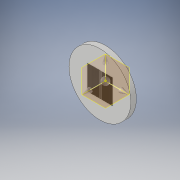
# Autodesk Inventor part: mask
Saved by Autodesk Inventor 2018 (Build 220112000, 112)
## iProperties
Created: 2019-06-01
Part Number: mask
Material: Generic
Document SubType Name: Modeling
Designer: 3esha
Density: 1 g/cm^3
Appearance: Default
Author: 3esha
Autodesk Inventor part; units mm, degrees
ref_plane "YZ Plane" through (0, 0, 0) normal (1, 0, 0) x (0, 1, 0)
ref_plane "XZ Plane" through (0, 0, 0) normal (0, 1, 0) x (-1, 0, 0)
ref_plane "XY Plane" through (0, 0, 0) normal (0, 0, 1) x (1, 0, 0)
sketch "Sketch9" plane through (0, 0, 0) normal (0, 0, 1) x (1, 0, 0)
  circle A0 centre (0, 0) radius 12.7
  line L0 (-0.3556, 4.953) -> (-0.4826, 4.953)
  line L1 (-0.4826, 4.953) -> (-0.4826, -5.0546)
  line L2 (-0.4826, -5.0546) -> (-0.3556, -5.0546)
  line L3 (-0.3556, -5.0546) -> (-0.3556, 4.953)
  line L4 (-0.635, 4.953) -> (-0.762, 4.953)
  line L5 (-0.762, 4.953) -> (-0.762, -5.0546)
  line L6 (-0.762, -5.0546) -> (-0.635, -5.0546)
  line L7 (-0.635, -5.0546) -> (-0.635, 4.953)
  line L8 (-0.889, 4.953) -> (-1.0414, 4.953)
  line L9 (-1.0414, 4.953) -> (-1.0414, -5.0546)
  line L10 (-1.0414, -5.0546) -> (-0.889, -5.0546)
  line L11 (-0.889, -5.0546) -> (-0.889, 4.953)
  line L12 (-1.1684, 4.953) -> (-1.2954, 4.953)
  line L13 (-1.2954, 4.953) -> (-1.2954, -5.0546)
  line L14 (-1.2954, -5.0546) -> (-1.1684, -5.0546)
  line L15 (-1.1684, -5.0546) -> (-1.1684, 4.953)
  line L16 (-1.4224, 4.953) -> (-1.5748, 4.953)
  line L17 (-1.5748, 4.953) -> (-1.5748, -5.0546)
  line L18 (-1.5748, -5.0546) -> (-1.4224, -5.0546)
  line L19 (-1.4224, -5.0546) -> (-1.4224, 4.953)
  line L20 (-1.7018, 4.953) -> (-1.8288, 4.953)
  line L21 (-1.8288, 4.953) -> (-1.8288, -5.0546)
  line L22 (-1.8288, -5.0546) -> (-1.7018, -5.0546)
  line L23 (-1.7018, -5.0546) -> (-1.7018, 4.953)
  line L24 (-1.9812, 4.953) -> (-2.1082, 4.953)
  line L25 (-2.1082, 4.953) -> (-2.1082, -5.0546)
  line L26 (-2.1082, -5.0546) -> (-1.9812, -5.0546)
  line L27 (-1.9812, -5.0546) -> (-1.9812, 4.953)
  line L28 (-2.2352, 4.953) -> (-2.3876, 4.953)
  line L29 (-2.3876, 4.953) -> (-2.3876, -5.0546)
  line L30 (-2.3876, -5.0546) -> (-2.2352, -5.0546)
  line L31 (-2.2352, -5.0546) -> (-2.2352, 4.953)
  line L32 (-2.5146, 4.953) -> (-2.6416, 4.953)
  line L33 (-2.6416, 4.953) -> (-2.6416, -5.0546)
  line L34 (-2.6416, -5.0546) -> (-2.5146, -5.0546)
  line L35 (-2.5146, -5.0546) -> (-2.5146, 4.953)
  line L36 (-2.794, 4.953) -> (-2.921, 4.953)
  line L37 (-2.921, 4.953) -> (-2.921, -5.0546)
  line L38 (-2.921, -5.0546) -> (-2.794, -5.0546)
  line L39 (-2.794, -5.0546) -> (-2.794, 4.953)
  line L40 (-3.048, 4.953) -> (-3.2004, 4.953)
  line L41 (-3.2004, 4.953) -> (-3.2004, -5.0546)
  line L42 (-3.2004, -5.0546) -> (-3.048, -5.0546)
  line L43 (-3.048, -5.0546) -> (-3.048, 4.953)
  line L44 (-3.3274, 4.953) -> (-3.4544, 4.953)
  line L45 (-3.4544, 4.953) -> (-3.4544, -5.0546)
  line L46 (-3.4544, -5.0546) -> (-3.3274, -5.0546)
  line L47 (-3.3274, -5.0546) -> (-3.3274, 4.953)
  line L48 (-3.6068, 4.953) -> (-3.7338, 4.953)
  line L49 (-3.7338, 4.953) -> (-3.7338, -5.0546)
  line L50 (-3.7338, -5.0546) -> (-3.6068, -5.0546)
  line L51 (-3.6068, -5.0546) -> (-3.6068, 4.953)
  line L52 (-3.8608, 4.953) -> (-3.9878, 4.953)
  line L53 (-3.9878, 4.953) -> (-3.9878, -5.0546)
  line L54 (-3.9878, -5.0546) -> (-3.8608, -5.0546)
  line L55 (-3.8608, -5.0546) -> (-3.8608, 4.953)
  line L56 (-4.1402, 4.953) -> (-4.2672, 4.953)
  line L57 (-4.2672, 4.953) -> (-4.2672, -5.0546)
  line L58 (-4.2672, -5.0546) -> (-4.1402, -5.0546)
  line L59 (-4.1402, -5.0546) -> (-4.1402, 4.953)
  line L60 (-4.3942, 4.953) -> (-4.5466, 4.953)
  line L61 (-4.5466, 4.953) -> (-4.5466, -5.0546)
  line L62 (-4.5466, -5.0546) -> (-4.3942, -5.0546)
  line L63 (-4.3942, -5.0546) -> (-4.3942, 4.953)
  line L64 (-4.6736, 4.953) -> (-4.8006, 4.953)
  line L65 (-4.8006, 4.953) -> (-4.8006, -5.0546)
  line L66 (-4.8006, -5.0546) -> (-4.6736, -5.0546)
  line L67 (-4.6736, -5.0546) -> (-4.6736, 4.953)
  line L68 (-4.953, 4.953) -> (-5.08, 4.953)
  line L69 (-5.08, 4.953) -> (-5.08, -5.0546)
  line L70 (-5.08, -5.0546) -> (-4.953, -5.0546)
  line L71 (-4.953, -5.0546) -> (-4.953, 4.953)
  line L72 (-0.0762, 4.953) -> (-0.2286, 4.953)
  line L73 (-0.2286, 4.953) -> (-0.2286, -5.0546)
  line L74 (-0.2286, -5.0546) -> (-0.0762, -5.0546)
  line L75 (-0.0762, -5.0546) -> (-0.0762, 4.953)
  line L76 (0.1778, 4.953) -> (0.3302, 4.953)
  line L77 (0.3302, 4.953) -> (0.3302, -5.0546)
  line L78 (0.3302, -5.0546) -> (0.1778, -5.0546)
  line L79 (0.1778, -5.0546) -> (0.1778, 4.953)
  line L80 (5.0546, 4.953) -> (5.1816, 4.953)
  line L81 (5.1816, 4.953) -> (5.1816, -5.0546)
  line L82 (5.1816, -5.0546) -> (5.0546, -5.0546)
  line L83 (5.0546, -5.0546) -> (5.0546, 4.953)
  line L84 (4.7752, 4.953) -> (4.9022, 4.953)
  line L85 (4.9022, 4.953) -> (4.9022, -5.0546)
  line L86 (4.9022, -5.0546) -> (4.7752, -5.0546)
  line L87 (4.7752, -5.0546) -> (4.7752, 4.953)
  line L88 (4.4958, 4.953) -> (4.6482, 4.953)
  line L89 (4.6482, 4.953) -> (4.6482, -5.0546)
  line L90 (4.6482, -5.0546) -> (4.4958, -5.0546)
  line L91 (4.4958, -5.0546) -> (4.4958, 4.953)
  line L92 (4.2418, 4.953) -> (4.3688, 4.953)
  line L93 (4.3688, 4.953) -> (4.3688, -5.0546)
  line L94 (4.3688, -5.0546) -> (4.2418, -5.0546)
  line L95 (4.2418, -5.0546) -> (4.2418, 4.953)
  line L96 (3.9624, 4.953) -> (4.0894, 4.953)
  line L97 (4.0894, 4.953) -> (4.0894, -5.0546)
  line L98 (4.0894, -5.0546) -> (3.9624, -5.0546)
  line L99 (3.9624, -5.0546) -> (3.9624, 4.953)
  line L100 (3.7084, 4.953) -> (3.8354, 4.953)
  line L101 (3.8354, 4.953) -> (3.8354, -5.0546)
  line L102 (3.8354, -5.0546) -> (3.7084, -5.0546)
  line L103 (3.7084, -5.0546) -> (3.7084, 4.953)
  line L104 (3.429, 4.953) -> (3.556, 4.953)
  line L105 (3.556, 4.953) -> (3.556, -5.0546)
  line L106 (3.556, -5.0546) -> (3.429, -5.0546)
  line L107 (3.429, -5.0546) -> (3.429, 4.953)
  line L108 (3.1496, 4.953) -> (3.302, 4.953)
  line L109 (3.302, 4.953) -> (3.302, -5.0546)
  line L110 (3.302, -5.0546) -> (3.1496, -5.0546)
  line L111 (3.1496, -5.0546) -> (3.1496, 4.953)
  line L112 (2.8956, 4.953) -> (3.0226, 4.953)
  line L113 (3.0226, 4.953) -> (3.0226, -5.0546)
  line L114 (3.0226, -5.0546) -> (2.8956, -5.0546)
  line L115 (2.8956, -5.0546) -> (2.8956, 4.953)
  line L116 (2.6162, 4.953) -> (2.7432, 4.953)
  line L117 (2.7432, 4.953) -> (2.7432, -5.0546)
  line L118 (2.7432, -5.0546) -> (2.6162, -5.0546)
  line L119 (2.6162, -5.0546) -> (2.6162, 4.953)
  line L120 (2.3368, 4.953) -> (2.4892, 4.953)
  line L121 (2.4892, 4.953) -> (2.4892, -5.0546)
  line L122 (2.4892, -5.0546) -> (2.3368, -5.0546)
  line L123 (2.3368, -5.0546) -> (2.3368, 4.953)
  line L124 (2.0828, 4.953) -> (2.2098, 4.953)
  line L125 (2.2098, 4.953) -> (2.2098, -5.0546)
  line L126 (2.2098, -5.0546) -> (2.0828, -5.0546)
  line L127 (2.0828, -5.0546) -> (2.0828, 4.953)
  line L128 (1.8034, 4.953) -> (1.9304, 4.953)
  line L129 (1.9304, 4.953) -> (1.9304, -5.0546)
  line L130 (1.9304, -5.0546) -> (1.8034, -5.0546)
  line L131 (1.8034, -5.0546) -> (1.8034, 4.953)
  line L132 (1.524, 4.953) -> (1.6764, 4.953)
  line L133 (1.6764, 4.953) -> (1.6764, -5.0546)
  line L134 (1.6764, -5.0546) -> (1.524, -5.0546)
  line L135 (1.524, -5.0546) -> (1.524, 4.953)
  line L136 (1.27, 4.953) -> (1.397, 4.953)
  line L137 (1.397, 4.953) -> (1.397, -5.0546)
  line L138 (1.397, -5.0546) -> (1.27, -5.0546)
  line L139 (1.27, -5.0546) -> (1.27, 4.953)
  line L140 (0.9906, 4.953) -> (1.143, 4.953)
  line L141 (1.143, 4.953) -> (1.143, -5.0546)
  line L142 (1.143, -5.0546) -> (0.9906, -5.0546)
  line L143 (0.9906, -5.0546) -> (0.9906, 4.953)
  line L144 (0.7366, 4.953) -> (0.8636, 4.953)
  line L145 (0.8636, 4.953) -> (0.8636, -5.0546)
  line L146 (0.8636, -5.0546) -> (0.7366, -5.0546)
  line L147 (0.7366, -5.0546) -> (0.7366, 4.953)
  line L148 (0.4572, 4.953) -> (0.5842, 4.953)
  line L149 (0.5842, 4.953) -> (0.5842, -5.0546)
  line L150 (0.5842, -5.0546) -> (0.4572, -5.0546)
  line L151 (0.4572, -5.0546) -> (0.4572, 4.953)
  line L152 (-5.08, 4.953) -> (-4.953, 4.953)
  line L153 (-4.953, 4.953) -> (-4.953, -5.0546)
  line L154 (-4.953, -5.0546) -> (-5.08, -5.0546)
  line L155 (-5.08, -5.0546) -> (-5.08, 4.953)
  line L156 (-4.8006, 4.953) -> (-4.6736, 4.953)
  line L157 (-4.6736, 4.953) -> (-4.6736, -5.0546)
  line L158 (-4.6736, -5.0546) -> (-4.8006, -5.0546)
  line L159 (-4.8006, -5.0546) -> (-4.8006, 4.953)
  line L160 (-4.2672, 4.953) -> (-4.1402, 4.953)
  line L161 (-4.1402, 4.953) -> (-4.1402, -5.0546)
  line L162 (-4.1402, -5.0546) -> (-4.2672, -5.0546)
  line L163 (-4.2672, -5.0546) -> (-4.2672, 4.953)
  line L164 (-3.9878, 4.953) -> (-3.8608, 4.953)
  line L165 (-3.8608, 4.953) -> (-3.8608, -5.0546)
  line L166 (-3.8608, -5.0546) -> (-3.9878, -5.0546)
  line L167 (-3.9878, -5.0546) -> (-3.9878, 4.953)
  line L168 (-3.7338, 4.953) -> (-3.6068, 4.953)
  line L169 (-3.6068, 4.953) -> (-3.6068, -5.0546)
  line L170 (-3.6068, -5.0546) -> (-3.7338, -5.0546)
  line L171 (-3.7338, -5.0546) -> (-3.7338, 4.953)
  line L172 (-3.4544, 4.953) -> (-3.3274, 4.953)
  line L173 (-3.3274, 4.953) -> (-3.3274, -5.0546)
  line L174 (-3.3274, -5.0546) -> (-3.4544, -5.0546)
  line L175 (-3.4544, -5.0546) -> (-3.4544, 4.953)
  line L176 (-3.2004, 4.953) -> (-3.048, 4.953)
  line L177 (-3.048, 4.953) -> (-3.048, -5.0546)
  line L178 (-3.048, -5.0546) -> (-3.2004, -5.0546)
  line L179 (-3.2004, -5.0546) -> (-3.2004, 4.953)
  line L180 (-2.921, 4.953) -> (-2.794, 4.953)
  line L181 (-2.794, 4.953) -> (-2.794, -5.0546)
  line L182 (-2.794, -5.0546) -> (-2.921, -5.0546)
  line L183 (-2.921, -5.0546) -> (-2.921, 4.953)
  line L184 (-2.6416, 4.953) -> (-2.5146, 4.953)
  line L185 (-2.5146, 4.953) -> (-2.5146, -5.0546)
  line L186 (-2.5146, -5.0546) -> (-2.6416, -5.0546)
  line L187 (-2.6416, -5.0546) -> (-2.6416, 4.953)
  line L188 (-2.3876, 4.953) -> (-2.2352, 4.953)
  line L189 (-2.2352, 4.953) -> (-2.2352, -5.0546)
  line L190 (-2.2352, -5.0546) -> (-2.3876, -5.0546)
  line L191 (-2.3876, -5.0546) -> (-2.3876, 4.953)
  line L192 (-2.1082, 4.953) -> (-1.9812, 4.953)
  line L193 (-1.9812, 4.953) -> (-1.9812, -5.0546)
  line L194 (-1.9812, -5.0546) -> (-2.1082, -5.0546)
  line L195 (-2.1082, -5.0546) -> (-2.1082, 4.953)
  line L196 (-1.8288, 4.953) -> (-1.7018, 4.953)
  line L197 (-1.7018, 4.953) -> (-1.7018, -5.0546)
  line L198 (-1.7018, -5.0546) -> (-1.8288, -5.0546)
  line L199 (-1.8288, -5.0546) -> (-1.8288, 4.953)
  line L200 (-1.5748, 4.953) -> (-1.4224, 4.953)
  line L201 (-1.4224, 4.953) -> (-1.4224, -5.0546)
  line L202 (-1.4224, -5.0546) -> (-1.5748, -5.0546)
  line L203 (-1.5748, -5.0546) -> (-1.5748, 4.953)
  line L204 (-1.2954, 4.953) -> (-1.1684, 4.953)
  line L205 (-1.1684, 4.953) -> (-1.1684, -5.0546)
  line L206 (-1.1684, -5.0546) -> (-1.2954, -5.0546)
  line L207 (-1.2954, -5.0546) -> (-1.2954, 4.953)
  line L208 (-1.0414, 4.953) -> (-0.889, 4.953)
  line L209 (-0.889, 4.953) -> (-0.889, -5.0546)
  line L210 (-0.889, -5.0546) -> (-1.0414, -5.0546)
  line L211 (-1.0414, -5.0546) -> (-1.0414, 4.953)
  line L212 (-0.762, 4.953) -> (-0.635, 4.953)
  line L213 (-0.635, 4.953) -> (-0.635, -5.0546)
  line L214 (-0.635, -5.0546) -> (-0.762, -5.0546)
  line L215 (-0.762, -5.0546) -> (-0.762, 4.953)
  line L216 (-0.4826, 4.953) -> (-0.3556, 4.953)
  line L217 (-0.3556, 4.953) -> (-0.3556, -5.0546)
  line L218 (-0.3556, -5.0546) -> (-0.4826, -5.0546)
  line L219 (-0.4826, -5.0546) -> (-0.4826, 4.953)
  line L220 (-0.2286, 4.953) -> (-0.0762, 4.953)
  line L221 (-0.0762, 4.953) -> (-0.0762, -5.0546)
  line L222 (-0.0762, -5.0546) -> (-0.2286, -5.0546)
  line L223 (-0.2286, -5.0546) -> (-0.2286, 4.953)
  line L224 (0.1778, 4.953) -> (0.3302, 4.953)
  line L225 (0.3302, 4.953) -> (0.3302, -5.0546)
  line L226 (0.3302, -5.0546) -> (0.1778, -5.0546)
  line L227 (0.1778, -5.0546) -> (0.1778, 4.953)
  line L228 (0.4572, 4.953) -> (0.5842, 4.953)
  line L229 (0.5842, 4.953) -> (0.5842, -5.0546)
  line L230 (0.5842, -5.0546) -> (0.4572, -5.0546)
  line L231 (0.4572, -5.0546) -> (0.4572, 4.953)
  line L232 (0.7366, 4.953) -> (0.8636, 4.953)
  line L233 (0.8636, 4.953) -> (0.8636, -5.0546)
  line L234 (0.8636, -5.0546) -> (0.7366, -5.0546)
  line L235 (0.7366, -5.0546) -> (0.7366, 4.953)
  line L236 (0.9906, 4.953) -> (1.143, 4.953)
  line L237 (1.143, 4.953) -> (1.143, -5.0546)
  line L238 (1.143, -5.0546) -> (0.9906, -5.0546)
  line L239 (0.9906, -5.0546) -> (0.9906, 4.953)
  line L240 (1.27, 4.953) -> (1.397, 4.953)
  line L241 (1.397, 4.953) -> (1.397, -5.0546)
  line L242 (1.397, -5.0546) -> (1.27, -5.0546)
  line L243 (1.27, -5.0546) -> (1.27, 4.953)
  line L244 (1.524, 4.953) -> (1.6764, 4.953)
  line L245 (1.6764, 4.953) -> (1.6764, -5.0546)
  line L246 (1.6764, -5.0546) -> (1.524, -5.0546)
  line L247 (1.524, -5.0546) -> (1.524, 4.953)
  line L248 (1.8034, 4.953) -> (1.9304, 4.953)
  line L249 (1.9304, 4.953) -> (1.9304, -5.0546)
  line L250 (1.9304, -5.0546) -> (1.8034, -5.0546)
  line L251 (1.8034, -5.0546) -> (1.8034, 4.953)
  line L252 (2.0828, 4.953) -> (2.2098, 4.953)
  line L253 (2.2098, 4.953) -> (2.2098, -5.0546)
  line L254 (2.2098, -5.0546) -> (2.0828, -5.0546)
  line L255 (2.0828, -5.0546) -> (2.0828, 4.953)
  line L256 (2.3368, 4.953) -> (2.4892, 4.953)
  line L257 (2.4892, 4.953) -> (2.4892, -5.0546)
  line L258 (2.4892, -5.0546) -> (2.3368, -5.0546)
  line L259 (2.3368, -5.0546) -> (2.3368, 4.953)
  line L260 (2.6162, 4.953) -> (2.7432, 4.953)
  line L261 (2.7432, 4.953) -> (2.7432, -5.0546)
  line L262 (2.7432, -5.0546) -> (2.6162, -5.0546)
  line L263 (2.6162, -5.0546) -> (2.6162, 4.953)
  line L264 (2.8956, 4.953) -> (3.0226, 4.953)
  line L265 (3.0226, 4.953) -> (3.0226, -5.0546)
  line L266 (3.0226, -5.0546) -> (2.8956, -5.0546)
  line L267 (2.8956, -5.0546) -> (2.8956, 4.953)
  line L268 (3.1496, 4.953) -> (3.302, 4.953)
  line L269 (3.302, 4.953) -> (3.302, -5.0546)
  line L270 (3.302, -5.0546) -> (3.1496, -5.0546)
  line L271 (3.1496, -5.0546) -> (3.1496, 4.953)
  line L272 (3.429, 4.953) -> (3.556, 4.953)
  line L273 (3.556, 4.953) -> (3.556, -5.0546)
  line L274 (3.556, -5.0546) -> (3.429, -5.0546)
  line L275 (3.429, -5.0546) -> (3.429, 4.953)
  line L276 (3.7084, 4.953) -> (3.8354, 4.953)
  line L277 (3.8354, 4.953) -> (3.8354, -5.0546)
  line L278 (3.8354, -5.0546) -> (3.7084, -5.0546)
  line L279 (3.7084, -5.0546) -> (3.7084, 4.953)
  line L280 (3.9624, 4.953) -> (4.0894, 4.953)
  line L281 (4.0894, 4.953) -> (4.0894, -5.0546)
  line L282 (4.0894, -5.0546) -> (3.9624, -5.0546)
  line L283 (3.9624, -5.0546) -> (3.9624, 4.953)
  line L284 (4.2418, 4.953) -> (4.3688, 4.953)
  line L285 (4.3688, 4.953) -> (4.3688, -5.0546)
  line L286 (4.3688, -5.0546) -> (4.2418, -5.0546)
  line L287 (4.2418, -5.0546) -> (4.2418, 4.953)
  line L288 (4.4958, 4.953) -> (4.6482, 4.953)
  line L289 (4.6482, 4.953) -> (4.6482, -5.0546)
  line L290 (4.6482, -5.0546) -> (4.4958, -5.0546)
  line L291 (4.4958, -5.0546) -> (4.4958, 4.953)
  line L292 (4.7752, 4.953) -> (4.9022, 4.953)
  line L293 (4.9022, 4.953) -> (4.9022, -5.0546)
  line L294 (4.9022, -5.0546) -> (4.7752, -5.0546)
  line L295 (4.7752, -5.0546) -> (4.7752, 4.953)
  line L296 (5.0546, 4.953) -> (5.1816, 4.953)
  line L297 (5.1816, 4.953) -> (5.1816, -5.0546)
  line L298 (5.1816, -5.0546) -> (5.0546, -5.0546)
  line L299 (5.0546, -5.0546) -> (5.0546, 4.953)
  line L300 (-4.5466, 4.953) -> (-4.3942, 4.953)
  line L301 (-4.3942, 4.953) -> (-4.3942, -5.0546)
  line L302 (-4.3942, -5.0546) -> (-4.5466, -5.0546)
  line L303 (-4.5466, -5.0546) -> (-4.5466, 4.953)
  constraints: 608 end point, 76 parallel, 38 horizontal, 38 perpendicular, 1 centre point, 1 coincident
extrude "Extrusion2" add sketch "Sketch9" along normal blind 2.286
body "Solid2"
